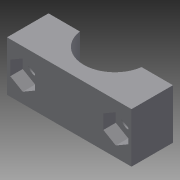
# Autodesk Inventor part: 8mm Rod clamp
Saved by Autodesk Inventor 2013 SP2 (Build 170200200, 200)
## iProperties
Created: 2017-03-11
Part Number: 8mm Rod clamp
Material: Generic
Document SubType Name: Modeling
Designer: Herman de Vries
Density: 1 g/cm^3
Author: Herman de Vries
Autodesk Inventor part; units mm, degrees
ref_plane "YZ Plane" through (0, 0, 0) normal (1, 0, 0) x (0, 1, 0)
ref_plane "XZ Plane" through (0, 0, 0) normal (0, 1, 0) x (-1, 0, 0)
ref_plane "XY Plane" through (0, 0, 0) normal (0, 0, 1) x (1, 0, 0)
sketch "Sketch1" plane through (0, 0, 0) normal (0, 0, 1) x (1, 0, 0)
  line L0 (0, 0) -> (30, 0)
  line L1 (30, 0) -> (30, 10)
  line L2 (30, 10) -> (0, 10) construction
  line L3 (0, 10) -> (0, 0)
  arc A0 (7.567, 10) -> (22.433, 10) centre (15, 11) ccw
  line L4 (0, 10) -> (7.567, 10)
  line L5 (22.433, 10) -> (30, 10)
  point P0 (15, 10)
  dimension "d0" = 30
  dimension "d1" = 10
  dimension "d2" = 15
  dimension "d3" = 1
  constraints: 12 end point, 2 collinear, 2 parallel, 2 point on circle, 2 point on line, 1 centre point, 1 horizontal, 1 midpoint, 1 perpendicular, 1 vertical alignment
  measures "d0" distance of L2.end L1.end
  measures "d1" distance of L0.end L1.end
  measures "d2" diameter of A0
  measures "d3" distance from line of L2 A0.centre
extrude "Extrusion1" add sketch "Sketch1" along normal blind 12
sketch "Sketch2" plane through (0, 10, 0) normal (0, 1, 0) x (1, 0, 0)
  line L0 (0, 0) -> (0, -12) construction
  line L1 (7.567, -12) -> (0, -12) construction
  line L2 (30, -12) -> (22.433, -12) construction
  circle A0 centre (3.7835, -6) radius 1.65
  circle A1 centre (26.2165, -6) radius 1.65
  point P0 (0, -6)
  point P1 (3.7835, -12)
  point P2 (26.2165, -12)
  dimension "d6" = 3.3
  dimension "d7" = 3.3
  constraints: 3 midpoint, 2 centre point, 2 horizontal alignment, 2 vertical alignment
  measures "d6" diameter of A0
  measures "d7" diameter of A1
extrude "Extrusion2" cut sketch "Sketch2" against normal blind 15
sketch "Sketch3" plane through (0, 0, 0) normal (0, -1, 0) x (1, 0, 0)
  circle A0 centre (3.7835, 6) radius 1.65 construction
  circle A1 centre (26.2165, 6) radius 1.65 construction
  line L0 (6.7835, 7.7321) -> (6.7835, 4.2679)
  line L1 (6.7835, 4.2679) -> (3.7835, 2.5359)
  line L2 (3.7835, 2.5359) -> (0.7835, 4.2679)
  line L3 (0.7835, 4.2679) -> (0.7835, 7.7321)
  line L4 (0.7835, 7.7321) -> (3.7835, 9.4641)
  line L5 (3.7835, 9.4641) -> (6.7835, 7.7321)
  line L6 (29.2165, 7.7321) -> (29.2165, 4.2679)
  line L7 (29.2165, 4.2679) -> (26.2165, 2.5359)
  line L8 (26.2165, 2.5359) -> (23.2165, 4.2679)
  line L9 (23.2165, 4.2679) -> (23.2165, 7.7321)
  line L10 (23.2165, 7.7321) -> (26.2165, 9.4641)
  line L11 (26.2165, 9.4641) -> (29.2165, 7.7321)
  point P0 (0, 0)
  dimension "d10" = 6
  dimension "d11" = 6
  constraints: 24 end point, 2 coincident, 2 vertical, 26 other
  measures "d10" distance between parallel lines of L0 L3
  measures "d11" distance between parallel lines of L6 L9
extrude "Extrusion3" cut sketch "Sketch3" against normal blind 3
equation "\"d6\" = d7"
body "Solid1"
